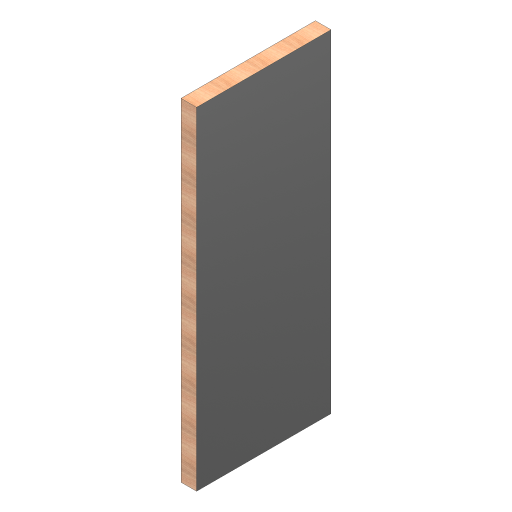
# Autodesk Inventor part: door
Saved by Autodesk Inventor 2023 (Build 270158000, 158)
## iProperties
Created: 2022-09-09
Part Number: door
Material: 木材(桦木)
Document SubType Name: Modeling
Designer: byfbi
Density: 0.55 g/cm^3
Appearance: 桦木 - 天然抛光
Author: byfbi
Autodesk Inventor part; units mm, degrees
ref_plane "YZ Plane" through (0, 0, 0) normal (1, 0, 0) x (0, 1, 0)
ref_plane "XZ Plane" through (0, 0, 0) normal (0, 1, 0) x (-1, 0, 0)
ref_plane "XY Plane" through (0, 0, 0) normal (0, 0, 1) x (1, 0, 0)
sketch "草图1" plane through (0, 0, 0) normal (1, 0, 0) x (0, 1, 0)
  line L0 (1175, -475) -> (-1175, -475)
  line L1 (-1175, -475) -> (-1175, 475)
  line L2 (-1175, 475) -> (1175, 475)
  line L3 (1175, 475) -> (1175, -475)
  line L4 (1175, -475) -> (-1175, 475) construction
  line L5 (-1175, -475) -> (1175, 475) construction
  point P0 (0, 0)
  dimension "d0" = 2350
  dimension "d1" = 950
  constraints: 12 end point, 2 midpoint, 2 parallel, 1 horizontal, 1 perpendicular
  measures "d0" distance of L1.end L2.end
  measures "d1" distance of L0.end L1.end
extrude "拉伸1" add sketch "草图1" along normal blind 110
